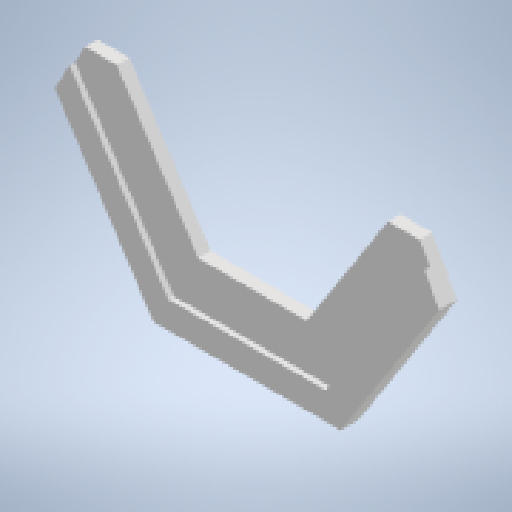
# Autodesk Inventor part: ДМС 045 держатель лотка
Saved by Autodesk Inventor 2024.2 (Build 282272000, 272)
## iProperties
Created: 2024-05-13
Part Number: ДМС 045 держатель лотка
Material: Generic
Document SubType Name: Modeling
Designer: admin
Density: 1 g/cm^3
Appearance: Default
Author: admin
Autodesk Inventor part; units mm, degrees
ref_plane "YZ Plane" through (0, 0, 0) normal (1, 0, 0) x (0, 1, 0)
ref_plane "XZ Plane" through (0, 0, 0) normal (0, 1, 0) x (-1, 0, 0)
ref_plane "XY Plane" through (0, 0, 0) normal (0, 0, 1) x (1, 0, 0)
sketch "Sketch1" plane through (0, 0, 0) normal (0, 1, 0) x (-1, 0, 0)
  line L0 (75, 70) -> (-75, 70) construction
  line L1 (-30, 0) -> (30, 0)
  line L2 (-30, 0) -> (-75, 70)
  line L3 (75, 70) -> (30, 0)
  line L4 (75, 70) -> (122.5523, 70)
  line L5 (122.5523, 70) -> (51.838, -40)
  line L6 (51.838, -40) -> (-51.838, -40)
  line L7 (-51.838, -40) -> (-122.5523, 70)
  line L8 (-122.5523, 70) -> (-75, 70)
  point P0 (0, 0)
  point P1 (0, 0)
  point P2 (0, 70)
  point P3 (0, -40)
  dimension "d0" = 150
  dimension "d1" = 60
  dimension "d2" = 70
  dimension "d3" = 40
  dimension "d5" = 40
  constraints: 18 end point, 3 horizontal, 3 midpoint, 3 parallel, 2 vertical alignment, 1 coincident, 1 collinear, 1 point on line
  measures "d0" distance of L0.start L0.end
  measures "d1" distance of L1.start L1.end
  measures "d2" distance between parallel lines of L1 L0
  measures "d3" distance between parallel lines of L6 L1
  measures "d5" distance between parallel lines of L5 L3
extrude "Extrusion1" add sketch "Sketch1" along normal blind 10
sketch "Sketch2" plane through (0, 0, 0) normal (0, -1, 0) x (1, 0, 0)
  line L0 (-30, 0) -> (30, 0) projected
  line L1 (-75, 70) -> (-30, 0) projected
  line L2 (-122.5523, 70) -> (-75, 70) projected
  line L3 (-51.838, -40) -> (-122.5523, 70) construction
  line L4 (51.838, -40) -> (-51.838, -40) construction
  line L5 (122.5523, 70) -> (51.838, -40) construction
  line L6 (75, 70) -> (122.5523, 70) projected
  line L7 (30, 0) -> (75, 70) projected
  line L8 (-98.7762, 70) -> (-40.919, -20)
  line L9 (-40.919, -20) -> (40.919, -20)
  line L10 (40.919, -20) -> (98.7762, 70)
  line L11 (75, 70) -> (122.5523, 70) projected
  line L12 (-75, 70) -> (-30, 0) projected
  line L13 (30, 0) -> (75, 70) projected
  point P0 (0, 0)
  dimension "d8" = 20
  dimension "d9" = 20
  dimension "d10" = 20
  constraints: 6 end point, 2 midpoint, 2 parallel, 1 horizontal
  measures "d8" distance between parallel lines of L9 L0
  measures "d9" distance between parallel lines of L1 L8
  measures "d10" distance between parallel lines of L7 L10
extrude "Extrusion2" cut sketch "Sketch2" against normal blind 3
chamfer "Chamfer1" distance 30 angle 45 2 edges at (122.5523, 5, 70) (-122.5523, 5, 70)
equation "\"d5\" = d3"
equation "\"d9\" = d8"
equation "\"d10\" = d8"
body "Solid1"
